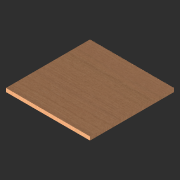
# Autodesk Inventor part: plate_wood_stabilizer
Saved by Autodesk Inventor 2020.3 (Build 243373010, 373A)
## iProperties
Created: 2021-04-14
Part Number: plate_wood_stabilizer
Material: Wood (Cherry)
Document SubType Name: Modeling
Designer: Melvin Strobl
Density: 0.63 g/cm^3
Appearance: Cherry - Natural Low Gloss
Author: Melvin Strobl
Autodesk Inventor part; units mm, degrees
ref_plane "YZ Plane" through (0, 0, 0) normal (1, 0, 0) x (0, 1, 0)
ref_plane "XZ Plane" through (0, 0, 0) normal (0, 1, 0) x (-1, 0, 0)
ref_plane "XY Plane" through (0, 0, 0) normal (0, 0, 1) x (1, 0, 0)
sketch "Sketch1" plane through (0, 0, 0) normal (0, 1, 0) x (-1, 0, 0)
  line L0 (0, 0) -> (236, 0)
  line L1 (236, 0) -> (236, -236)
  line L2 (236, -236) -> (0, -236)
  line L3 (0, -236) -> (0, 0)
  dimension "d0" = 236
  dimension "d1" = 236
  constraints: 8 end point, 2 parallel, 1 horizontal, 1 perpendicular
  measures "d0" distance of L1.end L2.end
  measures "d1" distance of L0.end L1.end
extrude "Extrusion1" add sketch "Sketch1" along normal blind 10
body "Solid1"
